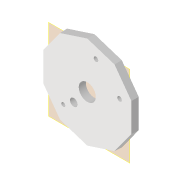
# Autodesk Inventor part: Anglerfish_Jar_Adapterplate_v1
Saved by Autodesk Inventor 2022 (Build 260153000, 153)
## iProperties
Created: 2022-04-02
Part Number: Anglerfish_Jar_Adapterplate_v1
Material: Generic
Document SubType Name: Modeling
Designer: Prakash Lab
Density: 1 g/cm^3
Appearance: Default
Author: Prakash Lab
Autodesk Inventor part; units mm, degrees
ref_plane "YZ Plane" through (0, 0, 0) normal (1, 0, 0) x (0, 1, 0)
ref_plane "XZ Plane" through (0, 0, 0) normal (0, 1, 0) x (-1, 0, 0)
ref_plane "XY Plane" through (0, 0, 0) normal (0, 0, 1) x (1, 0, 0)
ref_plane "Work Plane1" through (0, 0, 0) normal (0, 0, 1) x (1, 0, 0)
ref_plane "Arbeitsebene2" through (3.7631, 4.7567, 25.4) normal (0, 0, 1) x (1, 0, 0)
sketch "Skizze4" plane through (3.7631, 4.7567, 25.4) normal (0, 0, 1) x (1, 0, 0)
  circle A0 centre (0, 0) radius 25.9979 projected
  line L0 (31, -10.0725) -> (19.1591, -26.3702)
  line L1 (19.1591, -26.3702) -> (0, -32.5953)
  line L2 (0, -32.5953) -> (-19.1591, -26.3702)
  line L3 (-19.1591, -26.3702) -> (-31, -10.0725)
  line L4 (-31, -10.0725) -> (-31, 10.0725)
  line L5 (-31, 10.0725) -> (-19.1591, 26.3702)
  line L6 (-19.1591, 26.3702) -> (0, 32.5953)
  line L7 (0, 32.5953) -> (19.1591, 26.3702)
  line L8 (19.1591, 26.3702) -> (31, 10.0725)
  line L9 (31, 10.0725) -> (31, -10.0725)
  point P0 (-3.7631, -4.7567)
  point P1 (19.1591, 26.3702)
  point P2 (0, 32.5953)
  point P3 (-19.1591, -26.3702)
  point P4 (0, -32.5953)
  point P5 (31, -10.0725)
  dimension "d11" = 62
  constraints: 20 end point, 40 other
  measures "d11" distance between parallel lines of L4 L9
extrude "Extrusion4" add sketch "Skizze4" against normal blind 1 draft 2
ref_plane "Arbeitsebene3" through (3.7631, -5.3158, 913.1239) normal (1, 0, 0) x (0, 1, 0)
sketch "Skizze5" plane through (3.7631, -5.3158, 913.1239) normal (1, 0, 0) x (0, 1, 0)
  line L0 (-22.5228, -887.7239) -> (-22.5595, -888.7239) projected
  line L1 (-16.4204, -920.3789) -> (-16.4204, -919.8789)
  spline S0 degree 3 poles (2.3471, -919.6869) (-2.5417, -919.6399) (-6.9587, -919.5928) (-10.1713, -919.5458) (-13.3818, -919.4988) (-15.3766, -919.4518) (-15.8253, -919.4049) (-16.2764, -919.3576) (-15.162, -919.3104) (-12.6685, -919.2631) (-10.18, -919.216) (-6.3281, -919.1688) (-1.7554, -919.1217) (2.8097, -919.0746) (8.0747, -919.0275) (13.1646, -918.9804) (18.2473, -918.9334) (23.1349, -918.8864) (27.0172, -918.8394) (30.9167, -918.7922) (33.786, -918.745) (35.1453, -918.6978) (36.5, -918.6507) (36.35, -918.6037) (34.7204, -918.5566) (33.0872, -918.5095) (29.9742, -918.4623) (25.9005, -918.4152) (23.1924, -918.3838) (20.0707, -918.3525) (16.7723, -918.3211) knots 8.155694 8.155694 8.155694 8.155694 8.746524 8.746524 8.746524 9.336983 9.336983 9.336983 9.930706 9.930706 9.930706 10.523253 10.523253 10.523253 11.114793 11.114793 11.114793 11.705494 11.705494 11.705494 12.298807 12.298807 12.298807 12.890048 12.890048 12.890048 13.482595 13.482595 13.482595 13.876521 13.876521 13.876521 13.876521 projected
  spline S1 degree 3 poles (2.3471, -921.1869) (-2.5417, -921.1399) (-6.9587, -921.0928) (-10.1713, -921.0458) (-13.3818, -920.9988) (-15.3766, -920.9518) (-15.8253, -920.9049) (-16.2764, -920.8576) (-15.162, -920.8104) (-12.6685, -920.7631) (-10.18, -920.716) (-6.3281, -920.6688) (-1.7554, -920.6217) (2.8097, -920.5746) (8.0747, -920.5275) (13.1646, -920.4804) (18.2473, -920.4334) (23.1349, -920.3864) (27.0172, -920.3394) (30.9167, -920.2922) (33.786, -920.245) (35.1453, -920.1978) (36.5, -920.1507) (36.35, -920.1037) (34.7204, -920.0566) (33.0872, -920.0095) (29.9742, -919.9623) (25.9005, -919.9152) (23.1924, -919.8838) (20.0707, -919.8525) (16.7723, -919.8211) knots 1.872509 1.872509 1.872509 1.872509 2.463339 2.463339 2.463339 3.053798 3.053798 3.053798 3.647521 3.647521 3.647521 4.240067 4.240067 4.240067 4.831607 4.831607 4.831607 5.422309 5.422309 5.422309 6.015622 6.015622 6.015622 6.606863 6.606863 6.606863 7.19941 7.19941 7.19941 7.593336 7.593336 7.593336 7.593336 projected
  point P0 (5.3158, -913.1239)
  constraints: 2 end point, 1 vertical, 2 other
body "Solid1"
